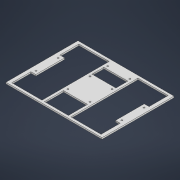
# Autodesk Inventor part: Testplatte_Differential
Saved by Autodesk Inventor 2021 (Build 250183000, 183)
## iProperties
Created: 2021-01-24
Part Number: Testplatte_Differential
Material: Generisch
Document SubType Name: Modeling
Designer: Ctroi
Density: 1 g/cm^3
Appearance: Vorgabe
Author: Ctroi
## iProperties of the stored document _3D-Druck.ipt
Created: 2021-01-30
Part Number: _3D-Druck
Material: Generisch
Document SubType Name: Modeling
Designer: Ctroi
Density: 1 g/cm^3
Appearance: Vorgabe
Author: Ctroi
Autodesk Inventor part; units mm, degrees
ref_plane "YZ Plane" through (0, 0, 0) normal (1, 0, 0) x (0, 1, 0)
ref_plane "XZ Plane" through (0, 0, 0) normal (0, 1, 0) x (-1, 0, 0)
ref_plane "XY Plane" through (0, 0, 0) normal (0, 0, 1) x (1, 0, 0)
sketch "Skizze1" plane through (0, 0, 0) normal (0, 1, 0) x (-1, 0, 0)
  line L0 (100, -75) -> (-100, -75)
  line L1 (-100, -75) -> (-100, 75)
  line L2 (-100, 75) -> (100, 75)
  line L3 (100, 75) -> (100, -75)
  line L4 (0, -105) -> (0, 105) projected
  line L5 (-140, 0) -> (140, 0) projected
  point P0 (0, 0)
  dimension "d0" = 200
  dimension "d1" = 150
  constraints: 8 end point, 2 parallel, 1 horizontal, 1 perpendicular, 2 other
  measures "d0" distance of L1.end L2.end
  measures "d1" distance of L0.end L1.end
extrude "Extrusion1" add sketch "Skizze1" along normal blind 3
sketch "Skizze11" plane through (0, 3, 0) normal (0, 1, 0) x (1, 0, 0)
  circle A0 centre (23, -23) radius 1.6
  circle A1 centre (23, 23) radius 1.6
  line L0 (140, 0) -> (-140, 0) projected
  line L1 (100, -75) -> (100, 75) projected
  line L2 (100, -75) -> (100, 75) projected
  line L3 (0, 105) -> (0, -105) projected
  circle A2 centre (-23, -23) radius 1.6
  circle A3 centre (-23, 23) radius 1.6
  circle A4 centre (23, 23) radius 1.6
  circle A5 centre (-23, 23) radius 1.6
  line L4 (100, 75) -> (-100, 75) projected
  circle A6 centre (89.5, -23) radius 1.6
  circle A7 centre (89.5, 23) radius 1.6
  circle A8 centre (-89.5, -23) radius 1.6
  circle A9 centre (-89.5, 23) radius 1.6
  line L5 (-100, 75) -> (-100, -75) projected
  point P0 (0, 0)
  dimension "d50" = 3.2
  dimension "d51" = 3.2
  dimension "d52" = 23
  dimension "d53" = 23
  dimension "d54" = 77
  dimension "d55" = 77
  dimension "d62" = 3.2
  dimension "d63" = 3.2
  dimension "d64" = 23
  dimension "d65" = 23
  dimension "d66" = 52
  dimension "d67" = 52
  dimension "d70" = 3.2
  dimension "d71" = 3.2
  dimension "d72" = 23
  dimension "d73" = 23
  dimension "d74" = 10.5
  dimension "d75" = 10.5
  dimension "d76" = 3.2
  dimension "d77" = 3.2
  dimension "d78" = 10.5
  dimension "d79" = 10.5
  dimension "d80" = 23
  dimension "d81" = 23
  constraints: 10 centre point, 2 symmetric about line, 2 other
  measures "d50" diameter of A0
  measures "d51" diameter of A1
  measures "d52" distance from line of L0 A0.centre
  measures "d53" distance from line of L0 A1.centre
  measures "d54" distance from line of L1 A1.centre
  measures "d55" distance from line of L2 A0.centre
  measures "d62" diameter of A4
  measures "d63" diameter of A5
  measures "d64" distance from line of L3 A4.centre
  measures "d65" distance from line of L3 A5.centre
  measures "d66" distance from line of L4 A5.centre
  measures "d67" distance from line of L4 A4.centre
  measures "d70" diameter of A6
  measures "d71" diameter of A7
  measures "d72" distance from line of L0 A6.centre
  measures "d73" distance from line of L0 A7.centre
  measures "d74" distance from line of L1 A6.centre
  measures "d75" distance from line of L1 A7.centre
  measures "d76" diameter of A8
  measures "d77" diameter of A9
  measures "d78" distance from line of L5 A9.centre
  measures "d79" distance from line of L5 A8.centre
  measures "d80" distance from line of L0 A8.centre
  measures "d81" distance from line of L0 A9.centre
extrude "Extrusion12" cut sketch "Skizze11" against normal up to surface (3 mm away) contours A0 | A1
extrude "Extrusion13" cut sketch "Skizze11" against normal up to surface (3 mm away) contours A2 | A3
extrude "Extrusion14" cut sketch "Skizze11" against normal up to surface (3 mm away) contours A1 | A3
extrude "Extrusion15" cut sketch "Skizze11" against normal up to surface (3 mm away) contours A6 | A7 | A8 | A9
sketch "Skizze12" plane through (0, 3, 0) normal (0, 1, 0) x (1, 0, 0)
  circle A0 centre (-23, 60) radius 1.6
  circle A1 centre (23, 60) radius 1.6
  line L0 (0, 105) -> (0, -105) projected
  line L1 (100, 75) -> (-100, 75) projected
  point P0 (0, 0)
  dimension "d84" = 3.2
  dimension "d85" = 3.2
  dimension "d86" = 23
  dimension "d87" = 23
  dimension "d88" = 15
  dimension "d89" = 15
  constraints: 2 centre point
  measures "d84" diameter of A0
  measures "d85" diameter of A1
  measures "d86" distance from line of L0 A1.centre
  measures "d87" distance from line of L0 A0.centre
  measures "d88" distance from line of L1 A1.centre
  measures "d89" distance from line of L1 A0.centre
extrude "Extrusion16" cut sketch "Skizze12" against normal up to surface (3 mm away)
sketch "Skizze13" plane through (0, 3, 0) normal (0, 1, 0) x (1, 0, 0)
  line L0 (-93, -70) -> (-30, -70)
  line L1 (-30, -70) -> (-30, 70)
  line L2 (-30, 70) -> (-93, 70)
  line L3 (30, -70) -> (93, -70)
  line L4 (93, 70) -> (30, 70)
  line L5 (30, 70) -> (30, -70)
  line L6 (-100, -75) -> (100, -75) projected
  line L7 (-100, 75) -> (-100, -75) projected
  line L8 (100, 75) -> (-100, 75) projected
  line L9 (100, -75) -> (100, 75) projected
  line L10 (-30, -70) -> (30, -70)
  line L11 (30, -70) -> (30, -30)
  line L12 (30, -30) -> (-30, -30)
  line L13 (-30, -30) -> (-30, -70)
  line L14 (-30, 29) -> (30, 29)
  line L15 (30, 29) -> (30, 54)
  line L16 (30, 54) -> (-30, 54)
  line L17 (-30, 54) -> (-30, 29)
  line L18 (-25, -70) -> (-25, -30)
  line L19 (25, -70) -> (25, -30)
  line L20 (-25, 29) -> (-25, 54)
  line L21 (25, 29) -> (25, 54)
  line L22 (-93, 30) -> (-83, 30)
  line L23 (-83, 30) -> (-83, -30)
  line L24 (-83, -30) -> (-93, -30)
  line L25 (140, 0) -> (-140, 0) projected
  line L26 (-93, 70) -> (-93, 30)
  line L27 (-93, -30) -> (-93, -70)
  line L28 (93, 30) -> (83, 30)
  line L29 (83, 30) -> (83, -30)
  line L30 (83, -30) -> (93, -30)
  line L31 (93, -70) -> (93, -30)
  line L32 (93, 30) -> (93, 70)
  point P0 (0, 0)
  dimension "d94" = 5
  dimension "d96" = 5
  dimension "d97" = 70
  dimension "d99" = 70
  dimension "d100" = 40
  dimension "d101" = 25
  dimension "d102" = 21
  dimension "d103" = 5
  dimension "d104" = 5
  dimension "d105" = 5
  dimension "d106" = 5
  dimension "d107" = 10
  dimension "d108" = 60
  dimension "d109" = 17
  dimension "d110" = 7
  dimension "d111" = 10
  dimension "d112" = 60
  dimension "d113" = 17
  dimension "d114" = 7
  constraints: 56 end point, 13 point on line, 12 parallel, 11 perpendicular, 6 horizontal, 2 other
  measures "d94" distance between parallel lines of L6 L0
  measures "d96" distance between parallel lines of L8 L2
  measures "d97" distance between parallel lines of L7 L1
  measures "d99" distance between parallel lines of L9 L5
  measures "d100" distance of L11.end L10.end
  measures "d101" distance of L15.end L14.end
  measures "d102" distance between parallel lines of L8 L16
  measures "d103" distance between parallel lines of L1 L18
  measures "d104" distance between parallel lines of L5 L19
  measures "d105" distance between parallel lines of L17 L20
  measures "d106" distance between parallel lines of L15 L21
  measures "d107" distance of L24.end L23.end
  measures "d108" distance of L22.end L23.end
  measures "d109" distance between parallel lines of L7 L23
  measures "d110" distance between parallel lines of L7 L26
  measures "d111" distance of L30.end L29.end
  measures "d112" distance of L29.end L28.end
  measures "d113" distance between parallel lines of L9 L29
  measures "d114" distance between parallel lines of L9 L32
extrude "Extrusion17" cut sketch "Skizze13" against normal up to surface (3 mm away) contours L27 L24 L23 L25 L1 L0 | L18 L12 L19 L10 | L25 L23 L22 L26 L2 L1 | L25 L29 L30 L31 L3 L5 | L5 L4 L32 L28 L29 L25 | L20 L16 L21 L14
